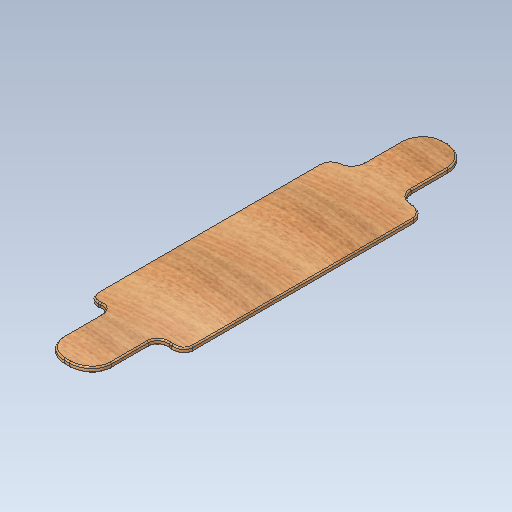
# Autodesk Inventor part: Skateboard Deck
Saved by Autodesk Inventor 2020 (Build 240168000, 168)
## iProperties
Created: 2019-01-13
Part Number: Skateboard Deck
Material: Generic
Document SubType Name: Modeling
Designer: LSabe
Density: 1 g/cm^3
Appearance: Default
Author: LSabe
Autodesk Inventor part; units mm, degrees
sketch "Sketch1" plane through (0, 0, 0) normal (0, 0, 1) x (1, 0, 0)
  line L0 (-73.66, 0) -> (-73.66, -12.8585)
  line L1 (154.94, 0) -> (154.94, -12.8585)
  arc A0 (-54.61, 2.7378) -> (-73.66, 0) centre (40.64, -727.6779) ccw
  arc A1 (154.94, 0) -> (-73.66, 0) centre (40.64, -727.6779) ccw
  arc A2 (154.94, -12.8585) -> (-73.66, -12.8585) centre (40.64, -727.6779) ccw
  point P0 (0, 0)
  dimension "d2" = 12.7
  constraints: 7 point on circle, 4 end point, 3 centre point
  measures "d2" radial gap between concentric circles of A1 A2
extrude "Extrusion1" add sketch "Sketch1" along normal blind 914.4
ref_plane "Center Long" through (40.64, -12.8585, 0) normal (-1, 0, 0) x (0, 0, 1)
ref_plane "Center Short" through (0, 0, 457.2) normal (0, 0, -1) x (-1, 0, 0)
ref_plane "Top Flat" through (0, 9.525, 0) normal (0, 1, 0) x (-1, 0, 0)
ref_plane "Right Oblique" through (154.94, 0, 0) normal (0.1551724, 0.9878874, 0) x (-0.9878874, 0.1551724, 0)
ref_plane "Left Oblique" through (-73.66, 0, 0) normal (-0.1551724, 0.9878874, 0) x (-0.9878874, -0.1551724, 0)
sketch "Sketch2" plane through (0, 9.525, 0) normal (0, 1, 0) x (-1, 0, 0)
  line L0 (73.66, 0) -> (-154.94, 0) projected
  line L1 (73.66, 0) -> (73.66, 914.4) projected
  line L2 (-154.94, 914.4) -> (73.66, 914.4) projected
  line L3 (-154.94, 0) -> (-154.94, 914.4) projected
  line L4 (73.66, 457.2) -> (-40.64, 457.2)
  line L5 (-40.64, 457.2) -> (-40.64, 203.2)
  line L6 (-40.64, 457.2) -> (-40.64, 711.2)
  line L7 (73.66, 914.4) -> (16.51, 914.4)
  line L8 (16.51, 914.4) -> (16.51, 749.3)
  line L9 (16.51, 749.3) -> (73.66, 749.3)
  line L10 (73.66, 749.3) -> (73.66, 914.4)
  line L11 (16.51, 914.4) -> (-97.79, 914.4)
  line L12 (-154.94, 914.4) -> (-97.79, 914.4)
  line L13 (-97.79, 914.4) -> (-97.79, 749.3)
  line L14 (-97.79, 749.3) -> (-154.94, 749.3)
  line L15 (-154.94, 749.3) -> (-154.94, 914.4)
  line L16 (-154.94, 0) -> (73.66, 0)
  line L17 (73.66, 0) -> (16.51, 0)
  line L18 (16.51, 0) -> (16.51, 165.1)
  line L19 (16.51, 165.1) -> (73.66, 165.1)
  line L20 (73.66, 165.1) -> (73.66, 0)
  line L21 (16.51, 0) -> (-97.79, 0)
  line L22 (-154.94, 0) -> (-97.79, 0)
  line L23 (-97.79, 0) -> (-97.79, 165.1)
  line L24 (-97.79, 165.1) -> (-154.94, 165.1)
  line L25 (-154.94, 165.1) -> (-154.94, 0)
  dimension "d6" = 254
  dimension "d8" = 254
  dimension "d19" = 165.1
  dimension "d20" = 57.15
  constraints: 44 end point, 9 symmetric about line, 2 parallel, 2 vertical, 1 collinear, 1 horizontal, 1 perpendicular
  measures "d6" distance of L4.end L5.end
  measures "d8" distance of L4.end L6.end
  measures "d19" distance of L7.end L8.end
  measures "d20" distance of L8.end L9.end
extrude "Extrusion2" cut sketch "Sketch2" against normal blind 50.8 contours L0 L18 L19 L1 | L0 L3 L24 L23 | L9 L8 L2 L1 | L3 L2 L13 L14
fillet "Fillet1" radius 25.4 8 edges at (-16.51, 0.3322, 749.3) (-73.66, -6.4292, 749.3) (97.79, 0.3322, 749.3) (154.94, -6.4292, 749.3) (-73.66, -6.4292, 165.1) (-16.51, 0.3322, 165.1) (97.79, 0.3322, 165.1) (154.94, -6.4292, 165.1)
fillet "Fillet2" radius 50.8 4 edges at (-16.51, 0.3322, 914.4) (97.79, 0.3322, 914.4) (-16.51, 0.3322, 0) (97.79, 0.3322, 0)
fillet "Fillet3" radius 3.175 48 edges at (126.3658, 3.9167, 165.1) (-45.0858, 3.9167, 165.1) (126.3658, 3.9167, 749.3) (-45.0858, 3.9167, 749.3) (103.938, 6.1974, 156.2687) (-23.065, 6.1622, 156.7302) (103.938, 6.1974, 758.1313) (-22.658, 6.1974, 758.1313) (97.79, 6.7018, 95.25) (-16.51, 6.7018, 95.25) (97.79, 6.7018, 819.15) (-16.51, 6.7018, 819.15) (84.6182, 7.6081, 897.7285) (-3.6656, 7.5885, 897.364) (40.64, 8.9221, 914.4) (-67.5859, 0.9281, 740.3824) (-73.66, 0, 457.2) (-67.5871, 0.928, 174.0191) (84.6182, 7.6081, 16.6715) (-3.6656, 7.5885, 17.036) (40.64, 8.9221, 0) (148.3781, 1.0004, 173.4623) (148.3781, 1.0004, 740.9377) (154.94, 0, 457.2) (154.94, -12.8585, 457.2) (148.8637, -11.9133, 174.015) (148.8637, -11.9133, 740.385) (126.3658, -8.8717, 165.1) (-45.0858, -8.8717, 165.1) (126.3658, -8.8717, 749.3) (-45.0858, -8.8717, 749.3) (103.9392, -6.5507, 156.27) (-23.0661, -6.5865, 156.7313) (103.9392, -6.5507, 758.13) (-22.6592, -6.5507, 758.13) (97.79, -6.0373, 95.25) (-16.51, -6.0373, 95.25) (97.79, -6.0373, 819.15) (-16.51, -6.0373, 819.15) (84.6183, -5.115, 16.6716) (-3.6656, -5.135, 17.0359) (40.64, -3.7779, 0) (-67.4819, -11.898, 173.8964) (-67.5851, -11.9136, 740.3833) (-73.66, -12.8585, 457.2) (-3.6656, -5.135, 897.3641) (40.64, -3.7779, 914.4) (84.6183, -5.115, 897.7284)
body "Solid1"
